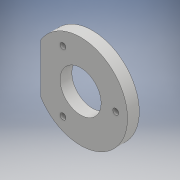
# Autodesk Inventor part: modified_o_ring
Saved by Autodesk Inventor 2018 (Build 220112000, 112)
## iProperties
Created: 2018-08-29
Part Number: modified_o_ring
Material: Generic
Document SubType Name: Modeling
Designer: David
Density: 1 g/cm^3
Appearance: Default
Author: David
Autodesk Inventor part; units mm, degrees
ref_plane "YZ Plane" through (0, 0, 0) normal (1, 0, 0) x (0, 1, 0)
ref_plane "XZ Plane" through (0, 0, 0) normal (0, 1, 0) x (-1, 0, 0)
ref_plane "XY Plane" through (0, 0, 0) normal (0, 0, 1) x (1, 0, 0)
sketch "Sketch1" plane through (0, 0, 0) normal (0, 1, 0) x (-1, 0, 0)
  circle A0 centre (0, 0) radius 8.75
  circle A1 centre (0, 0) radius 20
  dimension "d0" = 17.5
  dimension "d1" = 40
  constraints: 2 centre point, 2 coincident
  measures "d0" diameter of A0
  measures "d1" diameter of A1
extrude "Extrusion1" add sketch "Sketch1" along normal blind 5
sketch "Sketch2" plane through (0, 5, 0) normal (0, 1, 0) x (1, 0, 0)
  circle A0 centre (0, 0) radius 15 construction
  circle A1 centre (15, 0) radius 2.55
  circle A2 centre (0, 0) radius 15 construction
  circle A3 centre (-7.5, 12.9904) radius 2.55
  circle A4 centre (0, 0) radius 15 construction
  circle A5 centre (-7.5, -12.9904) radius 2.55
  dimension "d4" = 30
  dimension "d5" = 5.1
  dimension "d8" = 360
  constraints: 3 centre point, 1 coincident, 1 horizontal alignment, 21 other
  measures "d5" diameter of A1
extrude "Extrusion3" cut sketch "Sketch2" against normal blind 2
sketch "Sketch3" plane through (-7.5, 3, 12.9904) normal (0, 1, 0) x (1, 0, 0)
  circle A0 centre (0, 0) radius 1.25
  circle A1 centre (22.5, 12.9904) radius 2.55 projected
  circle A2 centre (22.5, 12.9904) radius 1.25
  circle A3 centre (0, 25.9808) radius 2.55 projected
  circle A4 centre (0, 25.9808) radius 1.25
  point P0 (7.5, 12.9904)
  dimension "d14" = 2.5
  dimension "d15" = 2.5
  dimension "d16" = 2.5
  constraints: 3 centre point, 2 coincident
  measures "d14" diameter of A0
  measures "d15" diameter of A2
  measures "d16" diameter of A4
extrude "Extrusion4" cut sketch "Sketch3" against normal blind 3 contours A0 | A2 | A4
sketch "Sketch4" plane through (0, 0, 0) normal (0, -1, 0) x (1, 0, 0)
  line L0 (-17, -45) -> (-17, 22) projected
  arc A0 (-17, 10.5357) -> (-17, -10.5357) centre (0, 0) ccw
  constraints: 2 point on circle, 2 point on line, 1 centre point, 1 coincident
extrude "Extrusion5" cut sketch "Sketch4" against normal blind 10
body "Solid1"
